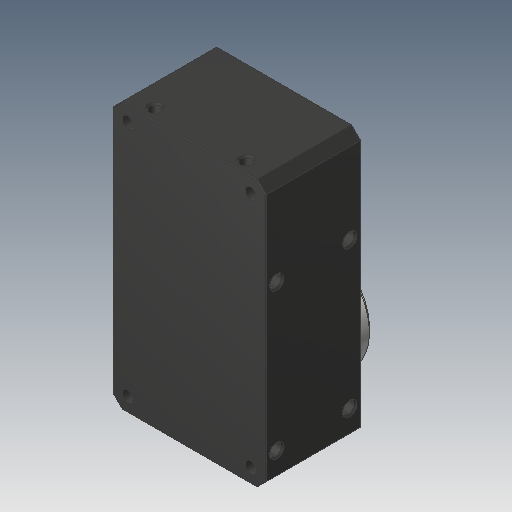
# Autodesk Inventor part: XM540_HOUSING_MIDDLE
Saved by Autodesk Inventor 2019.4 (Build 234330000, 330)
## iProperties
Created: 2019-10-19
Part Number: XM540_HOUSING_MIDDLE
Material: 一般
Document SubType Name: Modeling
Designer: y6tada
Density: 1 g/cm^3
Appearance: 滑らか - 黒
Mass: 25.045 g
Surface Area: 133.405 cm^2
Volume: 25.045 cm^3
Author: y6tada
Autodesk Inventor part; units mm, degrees
ref_plane "YZ Plane" through (0, 0, 0) normal (1, 0, 0) x (0, 1, 0)
ref_plane "XZ Plane" through (0, 0, 0) normal (0, 1, 0) x (-1, 0, 0)
ref_plane "XY Plane" through (0, 0, 0) normal (0, 0, 1) x (1, 0, 0)
sketch "スケッチ1" plane through (0, 0, 0) normal (0, 0, 1) x (1, 0, 0)
  line L0 (-14.75, 13.75) -> (14.75, 13.75)
  line L1 (16.75, 11.75) -> (16.75, -42.75)
  line L2 (14.75, -44.75) -> (-14.75, -44.75)
  line L3 (-16.75, -42.75) -> (-16.75, 11.75)
  line L4 (-14.75, 13.75) -> (-16.75, 11.75)
  line L5 (14.75, 13.75) -> (16.75, 11.75)
  line L6 (16.75, -42.75) -> (14.75, -44.75)
  line L7 (-14.75, -44.75) -> (-16.75, -42.75)
  line L8 (0, 0) -> (0, -49.9081) construction
  circle A0 centre (0, 0) radius 13 construction
  line L9 (-13.5, 10.5) -> (13.5, 10.5) construction
  line L10 (13.5, 10.5) -> (13.5, -41.5) construction
  line L11 (13.5, -41.5) -> (-13.5, -41.5) construction
  line L12 (-13.5, -41.5) -> (-13.5, 10.5) construction
  circle A1 centre (-13.5, 10.5) radius 1.25
  circle A2 centre (13.5, 10.5) radius 1.25
  circle A3 centre (13.5, -41.5) radius 1.25
  circle A4 centre (-13.5, -41.5) radius 1.25
  point P0 (-16.75, 13.75)
  point P1 (16.75, -44.75)
  point P2 (16.75, 13.75)
  point P3 (-16.75, -44.75)
  dimension "d0" = 2
  dimension "d1" = 2
  dimension "d2" = 2
  dimension "d3" = 2
  dimension "d4" = 2
  dimension "d5" = 2
  dimension "d6" = 2
  dimension "d7" = 2
  dimension "d8" = 33.5
  dimension "d9" = 26
  dimension "d10" = 13.75
  dimension "d11" = 58.5
  dimension "d24" = 27
  dimension "d25" = 10.5
  dimension "d26" = 52
  dimension "d27" = 2.5
  constraints: 26 end point, 8 point on line, 5 centre point, 5 coincident, 4 parallel, 3 equal radius, 2 horizontal, 2 perpendicular, 1 vertical, 2 other
  measures "d0" distance of L0.start point (-16.75, 13.75)
  measures "d1" distance of L3.end point (-16.75, 13.75)
  measures "d2" distance of L0.end point (16.75, 13.75)
  measures "d3" distance of L1.start point (16.75, 13.75)
  measures "d4" distance of L1.end point (16.75, -44.75)
  measures "d5" distance of L2.start point (16.75, -44.75)
  measures "d6" distance of L2.end point (-16.75, -44.75)
  measures "d7" distance of L3.start point (-16.75, -44.75)
  measures "d8" distance between parallel lines of L1 L3
  measures "d9" diameter of A0
  measures "d10" distance from line of L8.start L0
  measures "d11" distance between parallel lines of L2 L0
  measures "d24" distance of L9.start L9.end
  measures "d25" distance from line of A0.centre L9
  measures "d26" distance of L9.end L10.end
  measures "d27" diameter of A1
extrude "押し出し1" add sketch "スケッチ1" against normal blind 21
sketch "スケッチ6" plane through (16.75, -42.75, 0) normal (1, 0, 0) x (0, 0, -1)
  line L0 (0, 42.75) -> (40.1167, 42.75) construction
  line L1 (2.5, 36.75) -> (18.5, 36.75) construction
  line L2 (18.5, 36.75) -> (18.5, 4.75) construction
  line L3 (18.5, 4.75) -> (2.5, 4.75) construction
  line L4 (2.5, 4.75) -> (2.5, 36.75) construction
  line L5 (0, 56.5) -> (21, 56.5) construction
  line L6 (10.5, 56.5) -> (10.5, -5.6653) construction
  circle A0 centre (2.5, 36.75) radius 1.25
  circle A1 centre (18.5, 36.75) radius 1.25
  circle A2 centre (2.5, 4.75) radius 1.25
  circle A3 centre (18.5, 4.75) radius 1.25
  dimension "d48" = 16
  dimension "d49" = 6
  dimension "d50" = 32
  dimension "d51" = 2.5
  constraints: 12 end point, 4 centre point, 4 coincident, 3 equal radius, 2 horizontal, 2 parallel, 1 midpoint, 1 perpendicular, 1 vertical, 1 other
  measures "d48" distance of L1.start L1.end
  measures "d49" distance between parallel lines of L0 L1
  measures "d50" distance of L1.end L2.end
  measures "d51" diameter of A0
extrude "押し出し2" cut sketch "スケッチ6" against normal blind 3
sketch "スケッチ7" plane through (-14.75, 13.75, 0) normal (0, 1, 0) x (1, 0, 0)
  line L0 (14.75, 0) -> (14.75, 27.6085) construction
  circle A0 centre (24.75, 2.5) radius 1.25
  circle A1 centre (4.75, 2.5) radius 1.25
  dimension "d54" = 2.5
  dimension "d55" = 20
  dimension "d56" = 2.5
  constraints: 2 centre point, 2 end point, 1 symmetric about line, 1 vertical, 1 other
  measures "d54" diameter of A0
  measures "d55" distance of A0.centre A1.centre
  measures "d56" vertical distance of L0.start A0.centre
extrude "押し出し5" cut sketch "スケッチ7" against normal blind 3
sketch "スケッチ8" plane through (-14.75, -44.75, 0) normal (0, -1, 0) x (1, 0, 0)
  line L0 (14.75, 0) -> (14.75, -30.7913) construction
  circle A0 centre (24.75, -2.5) radius 1.25
  circle A1 centre (24.75, -18.5) radius 1.25
  line L1 (24.75, -2.5) -> (24.75, -18.5) construction
  line L2 (31.5, 0) -> (31.5, -21) construction
  line L3 (31.5, -10.5) -> (5.222, -10.5) construction
  circle A2 centre (4.75, -2.5) radius 1.25
  circle A3 centre (4.75, -18.5) radius 1.25
  dimension "d59" = 2.5
  dimension "d60" = 16
  dimension "d61" = 20
  constraints: 6 end point, 4 centre point, 3 symmetric about line, 2 vertical, 1 coincident, 1 equal radius, 1 horizontal, 1 midpoint, 2 other
  measures "d59" diameter of A0
  measures "d60" distance of L1.start L1.end
  measures "d61" diameter of L1 L0
extrude "押し出し6" cut sketch "スケッチ8" against normal blind 3
mirror "ミラー1" about plane through (0, 0, 0) normal (1, 0, 0) of "押し出し2"
sketch "スケッチ9" plane through (0, 0, -21) normal (0, 0, -1) x (-1, 0, 0)
  line L0 (14.75, 13.75) -> (-14.75, 13.75) construction
  line L1 (16.75, 11.75) -> (14.75, 13.75) construction
  line L2 (16.75, -42.75) -> (16.75, 11.75) construction
  line L3 (14.75, -44.75) -> (16.75, -42.75) construction
  line L4 (-14.75, -44.75) -> (14.75, -44.75) construction
  line L5 (-16.75, -42.75) -> (-14.75, -44.75) construction
  line L6 (-16.75, 11.75) -> (-16.75, -42.75) construction
  line L7 (-14.75, 13.75) -> (-16.75, 11.75) construction
  line L8 (-13.8387, 13.05) -> (13.8387, 13.05)
  line L9 (14.8994, 12.6107) -> (15.6107, 11.8994)
  line L10 (16.05, 10.8387) -> (16.05, -41.8387)
  line L11 (15.6107, -42.8994) -> (14.8994, -43.6107)
  line L12 (13.8387, -44.05) -> (-13.8387, -44.05)
  line L13 (-14.8994, -43.6107) -> (-15.6107, -42.8994)
  line L14 (-16.05, -41.8387) -> (-16.05, 10.8387)
  line L15 (-15.6107, 11.8994) -> (-14.8994, 12.6107)
  arc A0 (14.8994, 12.6107) -> (13.8387, 13.05) centre (13.8387, 11.55) ccw
  arc A1 (16.05, 10.8387) -> (15.6107, 11.8994) centre (14.55, 10.8387) ccw
  arc A2 (15.6107, -42.8994) -> (16.05, -41.8387) centre (14.55, -41.8387) ccw
  arc A3 (13.8387, -44.05) -> (14.8994, -43.6107) centre (13.8387, -42.55) ccw
  arc A4 (-14.8994, -43.6107) -> (-13.8387, -44.05) centre (-13.8387, -42.55) ccw
  arc A5 (-16.05, -41.8387) -> (-15.6107, -42.8994) centre (-14.55, -41.8387) ccw
  arc A6 (-15.6107, 11.8994) -> (-16.05, 10.8387) centre (-14.55, 10.8387) ccw
  arc A7 (-13.8387, 13.05) -> (-14.8994, 12.6107) centre (-13.8387, 11.55) ccw
  point P0 (0, 0)
  dimension "d64" = 0.7
  dimension "d65" = 1.5
  constraints: 16 end point, 16 point on circle, 16 tangent, 8 centre point, 7 equal radius, 7 other
  measures "d64" distance between parallel lines of L0 L8
  measures "d65" radius of A0
extrude "押し出し7" cut sketch "スケッチ9" against normal blind 0.8
sketch "スケッチ10" plane through (0, 0, -21) normal (0, 0, -1) x (-1, 0, 0)
  line L0 (-14.75, 13.75) -> (14.75, 13.75) construction
  line L1 (0, 13.75) -> (0, -44.75) construction
  line L2 (-14.75, -44.75) -> (14.75, -44.75) construction
  line L3 (-7, -43.35) -> (7, -43.35)
  line L4 (8.5, -41.85) -> (8.5, -39.55)
  line L5 (8.5, -39.55) -> (10.05, -39.55)
  line L6 (11.55, -38.05) -> (11.55, -36.75)
  line L7 (12.05, -36.25) -> (13.85, -36.25)
  line L8 (15.35, -34.75) -> (15.35, -26.22)
  line L9 (15.7, -23.5) -> (15.7, -10.5)
  line L10 (14.1191, -7.78) -> (12.05, -7.78)
  line L11 (11.55, -7.28) -> (11.55, -4.72)
  line L12 (12.05, -4.22) -> (13.85, -4.22)
  line L13 (15.35, -2.72) -> (15.35, 6.982)
  line L14 (-9.982, 12.35) -> (9.982, 12.35)
  line L15 (4.8838, -6) -> (31.9942, -6) construction
  arc A0 (11.482, 10.5) -> (13.5, 8.482) centre (13.5, 10.5) ccw
  circle A1 centre (13.5, 10.5) radius 1.25 construction
  line L16 (16.75, 11.75) -> (14.75, 13.75) construction
  line L17 (13.073, 8.073) -> (11.073, 10.073) construction
  line L18 (16.75, -42.75) -> (16.75, 11.75) construction
  line L19 (11.482, 10.5) -> (11.482, 10.85)
  line L20 (13.5, 8.482) -> (13.85, 8.482)
  arc A2 (15.35, -26.22) -> (15.7, -23.5) centre (4.9559, -23.5) ccw
  arc A3 (15.7, -10.5) -> (15.606, -9.082) centre (4.9559, -10.5) ccw
  arc A4 (12.05, -4.22) -> (11.55, -4.72) centre (12.05, -4.72) ccw
  arc A5 (11.55, -7.28) -> (12.05, -7.78) centre (12.05, -7.28) ccw
  arc A6 (12.05, -36.25) -> (11.55, -36.75) centre (12.05, -36.75) ccw
  arc A7 (7, -43.35) -> (8.5, -41.85) centre (7, -41.85) ccw
  arc A8 (10.05, -39.55) -> (11.55, -38.05) centre (10.05, -38.05) ccw
  arc A9 (13.85, -36.25) -> (15.35, -34.75) centre (13.85, -34.75) ccw
  arc A10 (15.606, -9.082) -> (14.1191, -7.78) centre (14.1191, -9.28) ccw
  arc A11 (13.85, -4.22) -> (15.35, -2.72) centre (13.85, -2.72) ccw
  arc A12 (15.35, 6.982) -> (13.85, 8.482) centre (13.85, 6.982) ccw
  arc A13 (11.482, 10.85) -> (9.982, 12.35) centre (9.982, 10.85) ccw
  line L21 (-8.5, -41.85) -> (-8.5, -39.55)
  line L22 (-8.5, -39.55) -> (-10.05, -39.55)
  line L23 (-11.55, -38.05) -> (-11.55, -36.75)
  line L24 (-12.05, -36.25) -> (-13.85, -36.25)
  line L25 (-15.35, -34.75) -> (-15.35, -26.22)
  line L26 (-15.7, -23.5) -> (-15.7, -10.5)
  line L27 (-14.1191, -7.78) -> (-12.05, -7.78)
  line L28 (-11.55, -7.28) -> (-11.55, -4.72)
  line L29 (-12.05, -4.22) -> (-13.85, -4.22)
  line L30 (-15.35, -2.72) -> (-15.35, 6.982)
  arc A14 (-13.5, 8.482) -> (-11.482, 10.5) centre (-13.5, 10.5) ccw
  line L31 (-11.482, 10.5) -> (-11.482, 10.85)
  line L32 (-13.5, 8.482) -> (-13.85, 8.482)
  arc A15 (-15.7, -23.5) -> (-15.35, -26.22) centre (-4.9559, -23.5) ccw
  arc A16 (-15.606, -9.082) -> (-15.7, -10.5) centre (-4.9559, -10.5) ccw
  arc A17 (-11.55, -4.72) -> (-12.05, -4.22) centre (-12.05, -4.72) ccw
  arc A18 (-12.05, -7.78) -> (-11.55, -7.28) centre (-12.05, -7.28) ccw
  arc A19 (-11.55, -36.75) -> (-12.05, -36.25) centre (-12.05, -36.75) ccw
  arc A20 (-8.5, -41.85) -> (-7, -43.35) centre (-7, -41.85) ccw
  arc A21 (-11.55, -38.05) -> (-10.05, -39.55) centre (-10.05, -38.05) ccw
  arc A22 (-15.35, -34.75) -> (-13.85, -36.25) centre (-13.85, -34.75) ccw
  arc A23 (-14.1191, -7.78) -> (-15.606, -9.082) centre (-14.1191, -9.28) ccw
  arc A24 (-15.35, -2.72) -> (-13.85, -4.22) centre (-13.85, -2.72) ccw
  arc A25 (-13.85, 8.482) -> (-15.35, 6.982) centre (-13.85, 6.982) ccw
  arc A26 (-9.982, 12.35) -> (-11.482, 10.85) centre (-9.982, 10.85) ccw
  point P0 (0, 0)
  point P1 (15.35, -7.78)
  point P2 (11.55, -7.78)
  point P3 (11.55, -4.22)
  point P4 (-15.35, -7.78)
  point P5 (-11.55, -7.78)
  point P6 (-11.55, -4.22)
  dimension "d68" = 6
  dimension "d69" = 3.56
  dimension "d71" = 5.2
  dimension "d72" = 1.4
  dimension "d73" = 1.4
  dimension "d75" = 5.2
  dimension "d76" = 1.05
  dimension "d77" = 24.25
  dimension "d78" = 13
  dimension "d80" = 1.4
  dimension "d81" = 8.5
  dimension "d82" = 5.2
  dimension "d83" = 5.2
  dimension "d84" = 8.25
  dimension "d85" = 0.5
  dimension "d86" = 1.5
  constraints: 58 end point, 54 point on circle, 42 symmetric about line, 26 centre point, 25 tangent, 14 point on line, 9 equal radius, 7 perpendicular, 4 horizontal, 2 midpoint, 1 concentric, 1 parallel, 1 vertical, 14 other
  measures "d68" distance from line of L15 point (0, 0)
  measures "d69" distance of point (11.55, -7.78) point (11.55, -4.22)
  measures "d71" distance between parallel lines of L16 L17
  measures "d72" distance between parallel lines of L18 L13
  measures "d73" distance between parallel lines of L0 L14
  measures "d75" distance between parallel lines of L18 L11
  measures "d76" distance between parallel lines of L18 L9
  measures "d77" distance from line of L9.end L0
  measures "d78" distance of L9.start L9.end
  measures "d80" distance between parallel lines of L3 L2
  measures "d81" distance between parallel lines of L2 L7
  measures "d82" distance between parallel lines of L18 L6
  measures "d83" distance between parallel lines of L2 L5
  measures "d84" distance between parallel lines of L18 L4
  measures "d85" radius of A4
  measures "d86" radius of A7
extrude "押し出し8" cut sketch "スケッチ10" against normal blind 16.65
chamfer "面取り3" distance 1 angle 45 1 edges at (-8.5, -39.55, -12.275)
sketch "スケッチ11" plane through (0, 0, -4.35) normal (0, 0, -1) x (-1, 0, 0)
  circle A0 centre (0.8, -31.25) radius 12
  line L0 (-3.9631, -43.25) -> (12.8, -43.25) construction
  line L1 (12.8, -43.25) -> (12.8, -16.7413) construction
  line L2 (16.75, -42.75) -> (16.75, 11.75) projected
  line L3 (-14.75, -44.75) -> (14.75, -44.75) projected
  point P0 (0, 0)
  dimension "d89" = 24
  dimension "d90" = 3.95
  dimension "d91" = 1.5
  constraints: 4 end point, 2 tangent, 1 centre point, 1 horizontal, 1 perpendicular
  measures "d89" diameter of A0
  measures "d90" distance between parallel lines of L2 L1
  measures "d91" distance between parallel lines of L3 L0
extrude "押し出し9" add sketch "スケッチ11" along normal blind 25
sketch "スケッチ12" plane through (-0.8, -31.25, -29.35) normal (0, 0, -1) x (-1, 0, 0)
  circle A0 centre (0, 0) radius 12 projected
  circle A1 centre (0, 0) radius 11
  point P0 (-0.8, 31.25)
  dimension "d94" = 1
  constraints: 1 centre point
  measures "d94" radial gap between concentric circles of A0 A1
extrude "押し出し10" cut sketch "スケッチ12" against normal blind 1
chamfer "面取り4" distance 0.2 angle 45 16 edges at (16.75, -15.5, 0) (15.75, 12.75, 0) (0, 13.75, 0) (-15.75, 12.75, 0) (-16.75, -15.5, 0) (-15.75, -43.75, 0) (0, -44.75, 0) (15.75, -43.75, 0) (-15.75, -43.75, -21) (0, -44.75, -21) (15.75, -43.75, -21) (16.75, -15.5, -21) (15.75, 12.75, -21) (0, 13.75, -21) (-15.75, 12.75, -21) (-16.75, -15.5, -21)
chamfer "面取り5" distance 0.325 angle 45 14 edges at (-16.75, -38, -1.25) (-16.75, -38, -17.25) (-11.25, -44.75, -18.5) (-11.25, -44.75, -2.5) (8.75, -44.75, -18.5) (8.75, -44.75, -2.5) (-16.75, -6, -1.25) (-16.75, -6, -17.25) (-11.25, 13.75, -2.5) (16.75, -38, -17.25) (16.75, -38, -1.25) (16.75, -6, -17.25) (16.75, -6, -1.25) (8.75, 13.75, -2.5)
equation "\"d1\" = d0"
equation "\"d2\" = d0"
equation "\"d3\" = d2"
equation "\"d4\" = d0"
equation "\"d5\" = d4"
equation "\"d6\" = d0"
equation "\"d7\" = d6"
